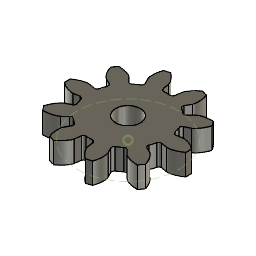
Spur Gear 2 (Autodesk Fusion 360 design; units mm, degrees)
part number: 2026-02-17-13-56-46-487
Autodesk Fusion 360 part; units mm, degrees
sketch "Base Circle" plane through (0, 0, 0) normal (0, 0, 1) x (1, 0, 0)
  circle A0 centre (0, 0) radius 7.686
  circle A1 centre (0, 0) radius 2.45
extrude "Extrude1" add sketch "Base Circle" along normal blind 4.2
sketch "Gear Tooth" plane through (0, 0, 0) normal (0, 0, 1) x (1, 0, 0)
  spline S0 degree 5 poles (9.2583, -1.6082) (9.2659, -1.6095) (9.2813, -1.6119) (9.3043, -1.6147) (9.3352, -1.6169) (9.374, -1.6176) (9.413, -1.6169) (9.4522, -1.6152) (9.4913, -1.6131) (9.5306, -1.6106) (9.5699, -1.6078) (9.6092, -1.6044) (9.6485, -1.6005) (9.688, -1.5957) (9.7275, -1.5903) (9.767, -1.5842) (9.8065, -1.5774) (9.8461, -1.5702) (9.8857, -1.5626) (9.9253, -1.5546) (9.9649, -1.5461) (10.0045, -1.5372) (10.0441, -1.5278) (10.0838, -1.5179) (10.1234, -1.5076) (10.163, -1.4969) (10.2027, -1.4857) (10.2423, -1.4741) (10.2819, -1.4621) (10.3215, -1.4497) (10.3611, -1.4369) (10.4006, -1.4237) (10.4402, -1.4102) (10.4797, -1.3962) (10.5192, -1.3819) (10.5587, -1.3672) (10.5982, -1.3521) (10.6376, -1.3367) (10.677, -1.3209) (10.7163, -1.3047) (10.7557, -1.2882) (10.795, -1.2713) (10.8342, -1.2541) (10.8734, -1.2366) (10.9126, -1.2187) (10.9517, -1.2004) (10.9908, -1.1818) (11.0298, -1.1629) (11.0688, -1.1437) (11.1078, -1.1241) (11.1466, -1.1042) (11.1855, -1.084) (11.2242, -1.0634) (11.2629, -1.0425) (11.3016, -1.0213) (11.3402, -0.9998) (11.3787, -0.978) (11.4172, -0.9559) (11.4556, -0.9334) (11.4939, -0.9107) (11.5322, -0.8876) (11.5704, -0.8642) (11.6085, -0.8406) (11.6466, -0.8166) (11.6846, -0.7923) (11.7225, -0.7677) (11.7603, -0.7429) (11.7981, -0.7177) (11.8358, -0.6923) (11.8733, -0.6665) (11.9109, -0.6405) (11.9408, -0.6194) (11.9632, -0.6035) (11.9781, -0.5928) (11.9856, -0.5875) knots 0 0 0 0 0 0 0.01428571 0.02857143 0.04285714 0.05714286 0.07142857 0.08571429 0.1 0.11428571 0.12857143 0.14285714 0.15714286 0.17142857 0.18571429 0.2 0.21428571 0.22857143 0.24285714 0.25714286 0.27142857 0.28571429 0.3 0.31428571 0.32857143 0.34285714 0.35714286 0.37142857 0.38571429 0.4 0.41428571 0.42857143 0.44285714 0.45714286 0.47142857 0.48571429 0.5 0.51428571 0.52857143 0.54285714 0.55714286 0.57142857 0.58571429 0.6 0.61428571 0.62857143 0.64285714 0.65714286 0.67142857 0.68571429 0.7 0.71428571 0.72857143 0.74285714 0.75714286 0.77142857 0.78571429 0.8 0.81428571 0.82857143 0.84285714 0.85714286 0.87142857 0.88571429 0.9 0.91428571 0.92857143 0.94285714 0.95714286 0.97142857 0.98571429 1 1 1 1 1 1
  spline S1 degree 5 poles (9.2583, 1.6082) (9.2659, 1.6095) (9.2813, 1.6119) (9.3043, 1.6147) (9.3352, 1.6169) (9.374, 1.6176) (9.413, 1.6169) (9.4522, 1.6152) (9.4913, 1.6131) (9.5306, 1.6106) (9.5699, 1.6078) (9.6092, 1.6044) (9.6485, 1.6005) (9.688, 1.5957) (9.7275, 1.5903) (9.767, 1.5842) (9.8065, 1.5774) (9.8461, 1.5702) (9.8857, 1.5626) (9.9253, 1.5546) (9.9649, 1.5461) (10.0045, 1.5372) (10.0441, 1.5278) (10.0838, 1.5179) (10.1234, 1.5076) (10.163, 1.4969) (10.2027, 1.4857) (10.2423, 1.4741) (10.2819, 1.4621) (10.3215, 1.4497) (10.3611, 1.4369) (10.4006, 1.4237) (10.4402, 1.4102) (10.4797, 1.3962) (10.5192, 1.3819) (10.5587, 1.3672) (10.5982, 1.3521) (10.6376, 1.3367) (10.677, 1.3209) (10.7163, 1.3047) (10.7557, 1.2882) (10.795, 1.2713) (10.8342, 1.2541) (10.8734, 1.2366) (10.9126, 1.2187) (10.9517, 1.2004) (10.9908, 1.1818) (11.0298, 1.1629) (11.0688, 1.1437) (11.1078, 1.1241) (11.1466, 1.1042) (11.1855, 1.084) (11.2242, 1.0634) (11.2629, 1.0425) (11.3016, 1.0213) (11.3402, 0.9998) (11.3787, 0.978) (11.4172, 0.9559) (11.4556, 0.9334) (11.4939, 0.9107) (11.5322, 0.8876) (11.5704, 0.8642) (11.6085, 0.8406) (11.6466, 0.8166) (11.6846, 0.7923) (11.7225, 0.7677) (11.7603, 0.7429) (11.7981, 0.7177) (11.8358, 0.6923) (11.8733, 0.6665) (11.9109, 0.6405) (11.9408, 0.6194) (11.9632, 0.6035) (11.9781, 0.5928) (11.9856, 0.5875) knots 0 0 0 0 0 0 0.01428571 0.02857143 0.04285714 0.05714286 0.07142857 0.08571429 0.1 0.11428571 0.12857143 0.14285714 0.15714286 0.17142857 0.18571429 0.2 0.21428571 0.22857143 0.24285714 0.25714286 0.27142857 0.28571429 0.3 0.31428571 0.32857143 0.34285714 0.35714286 0.37142857 0.38571429 0.4 0.41428571 0.42857143 0.44285714 0.45714286 0.47142857 0.48571429 0.5 0.51428571 0.52857143 0.54285714 0.55714286 0.57142857 0.58571429 0.6 0.61428571 0.62857143 0.64285714 0.65714286 0.67142857 0.68571429 0.7 0.71428571 0.72857143 0.74285714 0.75714286 0.77142857 0.78571429 0.8 0.81428571 0.82857143 0.84285714 0.85714286 0.87142857 0.88571429 0.9 0.91428571 0.92857143 0.94285714 0.95714286 0.97142857 0.98571429 1 1 1 1 1 1
  arc A0 (11.9856, -0.5875) -> (11.9856, 0.5875) centre (0, 0) ccw
  line L0 (7.5628, -1.3137) -> (9.2583, -1.6082)
  line L1 (7.5628, 1.3137) -> (9.2583, 1.6082)
  line L2 (7.5628, -1.3137) -> (7.5628, 1.3137)
  point P0 (9.4457, -1.6154)
  point P1 (9.6366, -1.6016)
  point P2 (9.8296, -1.5732)
  point P3 (10.0242, -1.5325)
  point P4 (10.2199, -1.4806)
  point P5 (10.4164, -1.4183)
  point P6 (10.6134, -1.3461)
  point P7 (10.8107, -1.2644)
  point P8 (11.008, -1.1735)
  point P9 (11.205, -1.0736)
  point P10 (11.4014, -0.9649)
  point P11 (11.5972, -0.8476)
  point P12 (11.792, -0.7217)
  point P13 (9.4457, 1.6154)
  point P14 (9.6366, 1.6016)
  point P15 (9.8296, 1.5732)
  point P16 (10.0242, 1.5325)
  point P17 (10.2199, 1.4806)
  point P18 (10.4164, 1.4183)
  point P19 (10.6134, 1.3461)
  point P20 (10.8107, 1.2644)
  point P21 (11.008, 1.1735)
  point P22 (11.205, 1.0736)
  point P23 (11.4014, 0.9649)
  point P24 (11.5972, 0.8476)
  point P25 (11.792, 0.7217)
extrude "Extrude2" add sketch "Gear Tooth" along normal blind 4.2
fillet "Fillet1" radius 0.5 2 edges at (7.5726, -1.3154, 2.1) (7.5726, 1.3154, 2.1)
pattern_circular "C-Pattern1" count 10 over 360 about axis through (0, 0, 0) along (0, 0, 1) of "Extrude2", "Fillet1"
sketch "Diametrial Pitch Circle" plane through (0, 0, 0) normal (0, 0, 1) x (1, 0, 0)
  circle A0 centre (0, 0) radius 10 construction
named bodies: "Spur Gear (10 teeth)"
